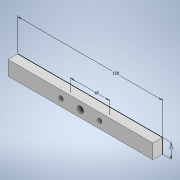
# Autodesk Inventor part: ParallelMecha_V2_BaseFormation_Proximal
Saved by Autodesk Inventor 2022 (Build 260153000, 153)
## iProperties
Created: 2022-08-03
Part Number: ParallelMecha_V2_BaseFormation_Proximal
Material: Generisch
Document SubType Name: Modeling
Designer: alexw
Density: 1 g/cm^3
Appearance: Vorgabe
Author: alexw
Autodesk Inventor part; units mm, degrees
ref_plane "YZ Plane" through (0, 0, 0) normal (1, 0, 0) x (0, 1, 0)
ref_plane "XZ Plane" through (0, 0, 0) normal (0, 1, 0) x (-1, 0, 0)
ref_plane "XY Plane" through (0, 0, 0) normal (0, 0, 1) x (1, 0, 0)
sketch "Skizze1" plane through (0, 0, 0) normal (0, 0, 1) x (1, 0, 0)
  line L0 (75, 7.5) -> (-75, 7.5)
  line L1 (-75, 7.5) -> (-75, -7.5)
  line L2 (-75, -7.5) -> (75, -7.5)
  line L3 (75, -7.5) -> (75, 7.5)
  line L4 (75, 7.5) -> (-75, -7.5) construction
  line L5 (-75, 7.5) -> (75, -7.5) construction
  line L6 (-20, 0) -> (20, 0) construction
  point P0 (0, 0)
  point P1 (0, 0)
  point P2 (0, 0)
  dimension "d0" = 40
  dimension "d1" = 15
  dimension "d2" = 150
  constraints: 14 end point, 4 midpoint, 2 horizontal, 2 parallel, 1 coincident, 1 perpendicular
  measures "d0" distance of L6.end L6.start
  measures "d1" distance between parallel lines of L0 L2
  measures "d2" distance between parallel lines of L3 L1
extrude "Extrusion1" add sketch "Skizze1" along normal blind 10
hole "Bohrung1" at (-20, 0, 0) at (20, 0, 0) direction (0, 0, 1) diameter 4.5 end through all clearance for "Inbusschraube DIN EN ISO 4762" size "M4" standard "DIN"
hole "Bohrung2" at (0, 0, 0) direction (0, 0, 1) diameter 6.6 end through all clearance for "Sechskantkopfschraube DIN EN 24017" size "M6" standard "DIN"
